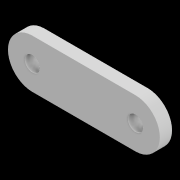
# Autodesk Inventor part: ForearmActuatorBracketLeft
Saved by Autodesk Inventor 2020 (Build 240168000, 168)
## iProperties
Created: 2020-04-15
Part Number: ForearmActuatorBracketLeft
Material: Generic
Document SubType Name: Modeling
Designer: valer
Density: 1 g/cm^3
Appearance: Default
Author: valer
Autodesk Inventor part; units mm, degrees
ref_plane "YZ Plane" through (0, 0, 0) normal (1, 0, 0) x (0, 1, 0)
ref_plane "XZ Plane" through (0, 0, 0) normal (0, 1, 0) x (-1, 0, 0)
ref_plane "XY Plane" through (0, 0, 0) normal (0, 0, 1) x (1, 0, 0)
sketch "Sketch1" plane through (0, 0, 0) normal (0, 0, 1) x (1, 0, 0)
  circle A0 centre (0, 0) radius 10.16
  line L0 (0, 10.16) -> (12.7, 10.16)
  line L1 (12.7, 10.16) -> (12.7, -10.16)
  line L2 (12.7, -10.16) -> (0, -10.16)
  line L3 (0, -10.16) -> (0, 10.16)
  circle A1 centre (0, 0) radius 3.175
  line L4 (12.7, 10.16) -> (27.7876, 10.16)
  line L5 (27.7876, 10.16) -> (27.7876, -10.16)
  line L6 (27.7876, -10.16) -> (12.7, -10.16)
  line L7 (12.7, -10.16) -> (12.7, 10.16)
  line L8 (27.7876, 10.16) -> (43.0276, 10.16)
  line L9 (43.0276, 10.16) -> (43.0276, -10.16)
  line L10 (43.0276, -10.16) -> (27.7876, -10.16)
  line L11 (27.7876, -10.16) -> (27.7876, 10.16)
  circle A2 centre (43.0276, 0) radius 10.16
  circle A3 centre (43.0276, 0) radius 3.175
  point P0 (0, -10.16)
  point P1 (12.7, -10.16)
  point P2 (43.0276, -10.16)
  dimension "d0" = 20.32
  dimension "d1" = 6.35
  dimension "d2" = 12.7
  dimension "d5" = 15.0876
  dimension "d6" = 15.24
  constraints: 24 end point, 6 parallel, 5 horizontal, 3 centre point, 3 perpendicular, 2 coincident, 2 collinear, 2 midpoint, 2 tangent, 1 equal radius, 3 other
  measures "d1" diameter of A1
  measures "d2" distance of L0.start L0.end
  measures "d5" distance of L0.end L4.end
  measures "d6" distance of L4.end L8.end
extrude "Extrusion1" add sketch "Sketch1" against normal blind 5.08 contours A0 L3 A1 | A0 L0 L1 L2 | L3 A1 A0 | L4 L5 L6 L1 | L8 A2 L10 L5 | A2 L9 A3 | L9 A3 A2
body "Solid1"
